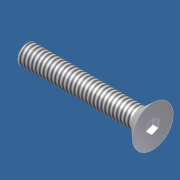
# Autodesk Inventor part: HW-00008
Saved by Autodesk Inventor 2012 (Build 160160000, 160)
## iProperties
Created: 2008-05-28
Part Number: HW-00008
Document SubType Name: Modeling
Designer: mcyr
Density: 1 g/cm^3
Description: FHCS 1/4-20 x 1.625"
Material: Default
Title: FHCS 1/4-20 x 1.625"
Author: mcyr
Autodesk Inventor part; units mm, degrees
ref_plane "YZ Plane" through (0, 0, 0) normal (1, 0, 0) x (0, 1, 0)
ref_plane "XZ Plane" through (0, 0, 0) normal (0, 1, 0) x (-1, 0, 0)
ref_plane "XY Plane" through (0, 0, 0) normal (0, 0, 1) x (1, 0, 0)
sketch "Sketch1" plane through (0, 0, 0) normal (0, 0, 1) x (1, 0, 0)
  line L0 (-11.9798, 0.1029) -> (29.2952, 0.1029)
  line L1 (29.2952, 0.1029) -> (29.2952, 6.8466)
  line L2 (29.2952, 6.8466) -> (25.2058, 3.2779)
  line L3 (25.2058, 3.2779) -> (-11.9798, 3.2779)
  line L4 (-11.9798, 3.2779) -> (-11.9798, 0.1029)
  dimension "d1" = 3.175
  dimension "d2" = 4.0894
  dimension "d3" = 6.7437
  dimension "d20" = 41.275
  constraints: 10 end point, 2 parallel, 1 horizontal, 1 perpendicular
  measures "d1" distance of L3.end L0.start
  measures "d2" horizontal distance of L1.end L2.end
  measures "d3" distance of L0.end L1.end
  measures "d20" distance of L0.start L0.end
revolve "Revolution1" add sketch "Sketch1" angle 360 about axis through (-11.9798, 0.1029, 0) along (1, 0, 0)
thread "Thread1" size "1/4-20 UNC" class "2A" standard "ANSI Unified Screw Threads" full length
sketch "Sketch2" plane through (29.2952, 0.1029, 0) normal (1, 0, 0) x (0, 0, -1)
  circle A0 centre (0, 0) radius 6.7437 projected
  line L0 (-1.8392, 1.3667) -> (0.264, 2.2761)
  line L1 (0.264, 2.2761) -> (2.1031, 0.9094)
  line L2 (2.1031, 0.9094) -> (1.8392, -1.3667)
  line L3 (1.8392, -1.3667) -> (-0.264, -2.2761)
  line L4 (-0.264, -2.2761) -> (-2.1031, -0.9094)
  line L5 (-2.1031, -0.9094) -> (-1.8392, 1.3667)
  dimension "d16" = 3.9688
  constraints: 12 end point, 1 coincident, 13 other
  measures "d16" distance between parallel lines of L2 L5
extrude "Extrusion1" cut sketch "Sketch2" against normal blind 1.905 contours L0 L1 L2 L3 L4 L5
body "Solid1"
